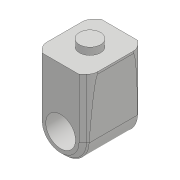
# Autodesk Inventor part: link4
Saved by Autodesk Inventor 2018 (Build 220112000, 112)
## iProperties
Created: 2018-02-01
Part Number: link4
Material: Generic
Document SubType Name: Modeling
Designer: Clevo
Density: 1 g/cm^3
Appearance: Default
Author: Clevo
Autodesk Inventor part; units mm, degrees
ref_plane "YZ Plane" through (0, 0, 0) normal (1, 0, 0) x (0, 1, 0)
ref_plane "XZ Plane" through (0, 0, 0) normal (0, 1, 0) x (-1, 0, 0)
ref_plane "XY Plane" through (0, 0, 0) normal (0, 0, 1) x (1, 0, 0)
sketch "Sketch1" plane through (0, 0, 0) normal (0, 1, 0) x (-1, 0, 0)
  line L0 (12.25, 22.5) -> (-12.25, 22.5)
  line L1 (-12.25, 22.5) -> (-12.25, -22.5)
  line L2 (-12.25, -22.5) -> (12.25, -22.5)
  line L3 (12.25, -22.5) -> (12.25, 22.5)
  point P0 (0, 0)
  point P1 (12.25, 0)
  point P2 (0, 22.5)
  dimension "d0" = 24.5
  dimension "d1" = 45
  constraints: 8 end point, 2 midpoint, 2 parallel, 1 horizontal, 1 horizontal alignment, 1 perpendicular, 1 vertical alignment
  measures "d0" distance of L2.end L1.end
  measures "d1" distance of L1.end L0.end
extrude "Extrusion1" add sketch "Sketch1" along normal blind 1.95
sketch "Sketch2" plane through (0, 1.95, 0) normal (0, 1, 0) x (1, 0, 0)
  line L0 (-10, 1.25) -> (10, 1.25)
  line L1 (10, 1.25) -> (10, -17.25)
  line L2 (10, -17.25) -> (-10, -17.25)
  line L3 (-10, -17.25) -> (-10, 1.25)
  line L4 (-12.25, -22.5) -> (12.25, -22.5) projected
  line L5 (12.25, -22.5) -> (12.25, 22.5) projected
  line L6 (12.25, 22.5) -> (-12.25, 22.5) projected
  line L7 (-12.25, 22.5) -> (-12.25, -22.5) projected
  line L8 (-7, -17.25) -> (7, -17.25)
  line L9 (7, -17.25) -> (7, -22.5)
  line L10 (7, -22.5) -> (-7, -22.5)
  line L11 (-7, -22.5) -> (-7, -17.25)
  line L12 (-12.25, -22.5) -> (12.25, -22.5) projected
  point P0 (0, 0)
  dimension "d4" = 2.25
  dimension "d5" = 20
  dimension "d6" = 2.25
  dimension "d7" = 5.25
  dimension "d8" = 5.25
  dimension "d9" = 14
  dimension "d10" = 5.25
  dimension "d11" = 18.5
  constraints: 16 end point, 4 parallel, 2 horizontal, 2 perpendicular, 1 collinear, 1 point on line
  measures "d4" distance between parallel lines of L7 L3
  measures "d5" distance of L0.start L0.end
  measures "d6" distance between parallel lines of L5 L1
  measures "d7" distance of L8.end L9.end
  measures "d8" distance between parallel lines of L7 L11
  measures "d9" distance between parallel lines of L9 L11
  measures "d10" distance between parallel lines of L5 L9
  measures "d11" distance of L0.end L1.end
extrude "Extrusion2" cut sketch "Sketch2" against normal up to surface (1.95 mm away) contours L0 L1 L2 L3 | L2 L9 L4 L11
sketch "Sketch3" plane through (0, 1.95, 0) normal (0, 1, 0) x (1, 0, 0)
  line L0 (-7, -22.5) -> (-7, -17.25) projected
  line L1 (-7, -17.25) -> (-10, -17.25) projected
  line L2 (-10, -17.25) -> (-10, 1.25) projected
  line L3 (-10, 1.25) -> (10, 1.25) projected
  line L4 (10, 1.25) -> (10, -17.25) projected
  line L5 (10, -17.25) -> (7, -17.25) projected
  line L6 (7, -17.25) -> (7, -22.5) projected
  line L7 (7, -22.5) -> (12.25, -22.5) projected
  line L8 (12.25, -22.5) -> (12.25, 22.5) projected
  line L9 (12.25, 22.5) -> (-12.25, 22.5) projected
  line L10 (-12.25, 22.5) -> (-12.25, -22.5) projected
  line L11 (-12.25, -22.5) -> (-7, -22.5) projected
  point P0 (0, 0)
  point P1 (-10.25, -20.305)
  point P2 (10.25, -20.305)
  dimension "d14" = 20.5
  dimension "d15" = 2
  dimension "d16" = 2.195
  dimension "d17" = 2
  constraints: 1 horizontal alignment
  measures "d14" distance of point (10.25, -20.305) point (-10.25, -20.305)
  measures "d15" distance from line of L8 point (10.25, -20.305)
  measures "d16" distance from line of L11 point (-10.25, -20.305)
  measures "d17" distance from line of L10 point (-10.25, -20.305)
hole "Hole1" at (-10.25, 1.95, 20.305) at (10.25, 1.95, 20.305) direction (0, -1, 0) diameter 2.4 end through all clearance for "Flat Head Machine Screw" size "M2" standard "Ansi Metric M Profile"
sketch "Sketch4" plane through (0, 1.95, 0) normal (0, 1, 0) x (1, 0, 0)
  circle A0 centre (-10.25, -20.305) radius 1.2 projected
  circle A1 centre (10.25, -20.305) radius 1.2 projected
  line L0 (-7, -22.5) -> (-7, -17.25) projected
  line L1 (-7, -17.25) -> (-10, -17.25) projected
  line L2 (-10, -17.25) -> (-10, 1.25) projected
  line L3 (-10, 1.25) -> (10, 1.25) projected
  line L4 (10, 1.25) -> (10, -17.25) projected
  line L5 (10, -17.25) -> (7, -17.25) projected
  line L6 (7, -17.25) -> (7, -22.5) projected
  line L7 (7, -22.5) -> (12.25, -22.5) projected
  line L8 (12.25, -22.5) -> (12.25, 22.5) projected
  line L9 (12.25, 22.5) -> (-12.25, 22.5) projected
  line L10 (-12.25, 22.5) -> (-12.25, -22.5) projected
  line L11 (-12.25, -22.5) -> (-7, -22.5) projected
  point P0 (0, 0)
  point P1 (-10.25, 4.15)
  point P2 (10.25, 4.15)
  dimension "d25" = 20.5
  dimension "d26" = 26.65
  dimension "d27" = 2
  dimension "d28" = 2
  constraints: 1 horizontal alignment
  measures "d25" distance of point (10.25, 4.15) point (-10.25, 4.15)
  measures "d26" distance from line of L11 point (-10.25, 4.15)
  measures "d27" distance from line of L10 point (-10.25, 4.15)
  measures "d28" distance from line of L8 point (10.25, 4.15)
hole "Hole2" at (-10.25, 1.95, -4.15) at (10.25, 1.95, -4.15) direction (0, -1, 0) diameter 2.4 end through all clearance for "Flat Head Machine Screw" size "M2" standard "Ansi Metric M Profile"
fillet "Fillet1" radius 0.5 2 edges at (7, 0.975, 17.25) (-7, 0.975, 17.25)
sketch "Sketch5" plane through (0, 1.95, 0) normal (0, 1, 0) x (1, 0, 0)
  circle A0 centre (-10.25, 4.15) radius 1.2 projected
  circle A1 centre (10.25, 4.15) radius 1.2 projected
  circle A2 centre (-10.25, -20.305) radius 1.2 projected
  circle A3 centre (10.25, -20.305) radius 1.2 projected
  arc A4 (-7, -17.75) -> (-7.5, -17.25) centre (-7.5, -17.75) ccw projected
  line L0 (-7.5, -17.25) -> (-10, -17.25) projected
  line L1 (-10, -17.25) -> (-10, 1.25) projected
  line L2 (-10, 1.25) -> (10, 1.25) projected
  line L3 (10, 1.25) -> (10, -17.25) projected
  line L4 (10, -17.25) -> (7.5, -17.25) projected
  arc A5 (7.5, -17.25) -> (7, -17.75) centre (7.5, -17.75) ccw projected
  line L5 (7, -17.75) -> (7, -22.5) projected
  line L6 (7, -22.5) -> (12.25, -22.5) projected
  line L7 (12.25, -22.5) -> (12.25, 22.5) projected
  line L8 (12.25, 22.5) -> (-12.25, 22.5) projected
  line L9 (-12.25, 22.5) -> (-12.25, -22.5) projected
  line L10 (-12.25, -22.5) -> (-7, -22.5) projected
  line L11 (-7, -22.5) -> (-7, -17.75) projected
  line L12 (-12.25, 22.5) -> (-12.25, -22.5) projected
  line L13 (12.25, -22.5) -> (12.25, 22.5) projected
  line L14 (-12.25, -22.5) -> (12.25, -22.5)
  line L15 (12.25, -22.5) -> (12.25, -4.5)
  line L16 (12.25, -4.5) -> (10, -4.5)
  line L17 (-12.25, -4.5) -> (-12.25, -22.5)
  line L18 (-10, -4.5) -> (-12.25, -4.5)
  line L19 (10, -4.5) -> (-10, -4.5)
  point P0 (0, 0)
  dimension "d37" = 18
  constraints: 12 end point, 4 parallel, 3 point on line, 1 horizontal, 1 perpendicular
  measures "d37" distance between parallel lines of L14 L16
extrude "Extrusion3" add sketch "Sketch5" along normal blind 5 contours L11 L10 L9 L18 L1 L0 A4 | A4 L0 L1 L19 L3 L4 A5 L5 L14 L11 | L5 A5 L4 L3 L16 L7 L6 | L18 L9 L8 L7 L16 L3 L2 L1
sketch "Sketch6" plane through (12.25, 0, 22.5) normal (1, 0, 0) x (0, 0, -1)
  line L0 (0, 0) -> (45, 0) projected
  line L1 (45, 0) -> (45, 6.95) projected
  line L2 (0, 6.95) -> (45, 6.95) projected
  line L3 (0, 0) -> (0, 6.95) projected
  line L4 (45, 0) -> (45, 6.95) projected
  line L5 (45, 6.95) -> (0, 6.95)
  line L6 (0, 6.95) -> (0, -32)
  line L7 (0, -32) -> (45, -32)
  line L8 (45, -32) -> (45, 6.95)
  line L9 (0, 0) -> (0, 6.95) projected
  line L10 (0, 0) -> (45, 0) projected
  line L11 (45, 0) -> (0, 0)
  line L12 (0, 0) -> (0, -32)
  line L13 (0, -32) -> (45, -32)
  line L14 (45, -32) -> (45, 0)
  point P0 (22.5, 0)
  dimension "d72" = 32
  constraints: 16 end point, 4 parallel, 2 horizontal, 2 perpendicular, 1 collinear
  measures "d72" distance between parallel lines of L0 L7
extrude "Extrusion4" add sketch "Sketch6" along normal blind 10
sketch "Sketch7" plane through (12.25, -32, -22.5) normal (0, -1, 0) x (1, 0, 0)
  line L0 (0, 45) -> (0, 0) projected
  line L1 (0, 0) -> (10, 0) projected
  line L2 (10, 45) -> (10, 0) projected
  line L3 (0, 45) -> (10, 45) projected
  line L4 (0, 0) -> (-24.5, 0) projected
  line L5 (0, 0) -> (-24.5, 0)
  line L6 (-24.5, 0) -> (-24.5, 45)
  line L7 (-24.5, 45) -> (0, 45)
  line L8 (0, 45) -> (0, 0)
  point P0 (-12.25, 22.5)
  dimension "d43" = 24.5
  constraints: 8 end point, 2 parallel, 1 collinear, 1 horizontal, 1 perpendicular
  measures "d43" distance of L0.end L5.end
extrude "Extrusion5" add sketch "Sketch7" along normal blind 1.15
sketch "Sketch8" plane through (12.25, -33.15, -22.5) normal (0, -1, 0) x (1, 0, 0)
  line L0 (-24.5, 0) -> (10, 0) projected
  line L1 (10, 0) -> (10, 45) projected
  line L2 (10, 45) -> (-24.5, 45) projected
  line L3 (-24.5, 45) -> (-24.5, 0) projected
  circle A0 centre (-12.25, 10) radius 10.5
  line L4 (-19.25, 45) -> (-5.25, 45) projected
  line L5 (-5, 45) -> (-19.5, 45)
  line L6 (-19.5, 45) -> (-19.5, 36)
  line L7 (-19.5, 36) -> (-5, 36)
  line L8 (-5, 36) -> (-5, 45)
  line L9 (-2.25, 21.25) -> (-22.25, 21.25)
  line L10 (-22.25, 21.25) -> (-22.25, 36)
  line L11 (-22.25, 36) -> (-2.25, 36)
  line L12 (-2.25, 36) -> (-2.25, 21.25)
  line L13 (-5, 21.25) -> (-19.5, 21.25)
  line L14 (-19.5, 21.25) -> (-19.5, 17.25)
  line L15 (-19.5, 17.25) -> (-5, 17.25)
  line L16 (-5, 17.25) -> (-5, 21.25)
  line L17 (-24.5, 0) -> (10, 0) projected
  line L18 (-24.5, 45) -> (0, 45)
  line L19 (0, 45) -> (0, 0)
  line L20 (0, 0) -> (-24.5, 0)
  line L21 (-24.5, 0) -> (-24.5, 45)
  point P0 (-12.25, 22.5)
  dimension "d46" = 10
  dimension "d47" = 21
  dimension "d48" = 14.5
  dimension "d49" = 20
  dimension "d50" = 14.5
  dimension "d51" = 24.5
  dimension "d52" = 5
  dimension "d53" = 5
  dimension "d54" = 2.25
  dimension "d55" = 2.25
  dimension "d56" = 5
  dimension "d57" = 5
  dimension "d58" = 9
  dimension "d59" = 14.75
  dimension "d60" = 4
  constraints: 32 end point, 8 parallel, 4 horizontal, 4 perpendicular, 4 point on line, 1 centre point, 1 vertical alignment
  measures "d46" distance from line of L0 A0.centre
  measures "d47" diameter of A0
  measures "d48" distance between parallel lines of L6 L8
  measures "d49" distance of L10.end L11.end
  measures "d50" distance of L14.end L15.end
  measures "d51" distance between parallel lines of L3 L19
  measures "d52" distance between parallel lines of L19 L16
  measures "d53" distance between parallel lines of L3 L14
  measures "d54" distance between parallel lines of L19 L12
  measures "d55" distance between parallel lines of L3 L10
  measures "d56" distance between parallel lines of L3 L6
  measures "d57" distance between parallel lines of L19 L8
  measures "d58" distance of L5.end L6.end
  measures "d59" distance of L9.end L10.end
  measures "d60" distance of L13.end L14.end
extrude "Extrusion6" cut sketch "Sketch8" against normal up to surface (1.15 mm away) contours A0 L0 | L0 A0 L14 L15 L16 | L8 L7 L6 L2 | L14 L9 L16 A0 | A0 L16 L15 L14 | L11 L12 L9 L10 L7
sketch "Sketch9" plane through (12.25, -33.15, -22.5) normal (0, -1, 0) x (1, 0, 0)
  line L0 (-5, 45) -> (-5, 36) projected
  line L1 (-5, 36) -> (-2.25, 36) projected
  line L2 (-2.25, 36) -> (-2.25, 21.25) projected
  line L3 (-2.25, 21.25) -> (-5, 21.25) projected
  line L4 (-5, 21.25) -> (-5, 17.5952) projected
  arc A0 (-9.0484, 0) -> (-5, 17.5952) centre (-12.25, 10) ccw projected
  line L5 (-9.0484, 0) -> (10, 0) projected
  line L6 (10, 0) -> (10, 45) projected
  line L7 (10, 45) -> (-5, 45) projected
  line L8 (-19.5, 36) -> (-19.5, 45) projected
  line L9 (-19.5, 45) -> (-24.5, 45) projected
  line L10 (-24.5, 45) -> (-24.5, 0) projected
  line L11 (-24.5, 0) -> (-15.4516, 0) projected
  arc A1 (-19.5, 17.5952) -> (-15.4516, 0) centre (-12.25, 10) ccw projected
  line L12 (-19.5, 17.5952) -> (-19.5, 21.25) projected
  line L13 (-19.5, 21.25) -> (-22.25, 21.25) projected
  line L14 (-22.25, 21.25) -> (-22.25, 36) projected
  line L15 (-22.25, 36) -> (-19.5, 36) projected
  circle A2 centre (-22.5, 18.35) radius 1.2 projected
  circle A3 centre (-2, 18.35) radius 1.2 projected
  circle A4 centre (-2, 42.805) radius 1.2 projected
  circle A5 centre (-22.5, 42.805) radius 1.2 projected
  line L16 (-2, 18.35) -> (-22.5, 18.35)
  line L17 (-22.5, 18.35) -> (-22.5, 39.05)
  line L18 (-22.5, 39.05) -> (-2, 39.05)
  line L19 (-2, 39.05) -> (-2, 18.35)
  point P0 (-12.25, 22.5)
  dimension "d63" = 20.7
  constraints: 8 end point, 2 parallel, 1 horizontal, 1 perpendicular, 1 point on line
  measures "d63" distance of L16.end L17.end
hole "Hole3" at (-10.25, -33.15, -4.15) at (10.25, -33.15, -4.15) at (10.25, -33.15, 16.55) at (-10.25, -33.15, 16.55) direction (0, 1, 0) diameter 2.4 depth 8 tip angle 118 clearance for "Flat Head Machine Screw" size "M2" standard "Ansi Metric M Profile"
sketch "Sketch10" plane through (12.25, -33.15, -22.5) normal (0, -1, 0) x (1, 0, 0)
  circle A0 centre (-2, 39.05) radius 1.2 projected
  circle A1 centre (-2, 18.35) radius 1.2 projected
  line L0 (-5, 45) -> (-5, 36) projected
  line L1 (-5, 36) -> (-2.25, 36) projected
  line L2 (-2.25, 36) -> (-2.25, 21.25) projected
  line L3 (-2.25, 21.25) -> (-5, 21.25) projected
  line L4 (-5, 21.25) -> (-5, 17.5952) projected
  arc A2 (-9.0484, 0) -> (-5, 17.5952) centre (-12.25, 10) ccw projected
  line L5 (-9.0484, 0) -> (10, 0) projected
  line L6 (10, 0) -> (10, 45) projected
  line L7 (10, 45) -> (-5, 45) projected
  circle A3 centre (-22.5, 18.35) radius 1.2 projected
  circle A4 centre (-22.5, 39.05) radius 1.2 projected
  line L8 (-19.5, 36) -> (-19.5, 45) projected
  line L9 (-19.5, 45) -> (-24.5, 45) projected
  line L10 (-24.5, 45) -> (-24.5, 0) projected
  line L11 (-24.5, 0) -> (-15.4516, 0) projected
  arc A5 (-19.5, 17.5952) -> (-15.4516, 0) centre (-12.25, 10) ccw projected
  line L12 (-19.5, 17.5952) -> (-19.5, 21.25) projected
  line L13 (-19.5, 21.25) -> (-22.25, 21.25) projected
  line L14 (-22.25, 21.25) -> (-22.25, 36) projected
  line L15 (-22.25, 36) -> (-19.5, 36) projected
  line L16 (10, 0) -> (10, 45) projected
  line L17 (-24.5, 0) -> (-24.5, 45) projected
  line L18 (10, 0) -> (-24.5, 0)
  line L19 (-24.5, 0) -> (-24.5, 45)
  line L20 (-24.5, 45) -> (10, 45)
  line L21 (10, 45) -> (10, 0)
  arc A6 (-19.5, 17.5952) -> (-15.4516, 0) centre (-12.25, 10) ccw projected
  circle A7 centre (-12.25, 10) radius 10.5
  point P0 (-12.25, 22.5)
  constraints: 8 end point, 2 parallel, 1 coincident, 1 horizontal, 1 perpendicular, 3 other
extrude "Extrusion7" add sketch "Sketch10" along normal blind 5
sketch "Sketch11" plane through (12.25, -38.15, -22.5) normal (0, -1, 0) x (1, 0, 0)
  line L0 (-9.0484, 0) -> (10, 0) projected
  line L1 (10, 0) -> (10, 45) projected
  line L2 (10, 45) -> (-24.5, 45) projected
  line L3 (-24.5, 45) -> (-24.5, 0) projected
  line L4 (-24.5, 0) -> (-15.4516, 0) projected
  arc A0 (-15.4516, 0) -> (-9.0484, 0) centre (-12.25, 10) ccw projected
  arc A1 (-19.5, 17.5952) -> (-15.4516, 0) centre (-12.25, 10) ccw projected
  circle A2 centre (-12.25, 10) radius 10.5
  point P0 (-12.25, 22.5)
  constraints: 1 coincident, 3 other
extrude "Extrusion8" cut sketch "Sketch11" against normal up to surface (5 mm away) contours A0 A1 A2
sketch "Sketch12" plane through (-12.25, 0, -22.5) normal (-1, 0, 0) x (0, 0, 1)
  line L0 (-6.0754, -39.5109) -> (50.3226, -39.5109)
  line L1 (50.3226, -39.5109) -> (50.3226, 16.733)
  line L2 (50.3226, 16.733) -> (-6.0754, 16.733)
  line L3 (-6.0754, 16.733) -> (-6.0754, -39.5109)
  point P0 (22.5, 0)
  constraints: 8 end point, 2 parallel, 1 horizontal, 1 perpendicular
extrude "Extrusion9" cut sketch "Sketch12" against normal blind 12.25
sketch "Sketch13" plane through (0, 0, 0) normal (0, -1, 0) x (1, 0, 0)
  arc A0 (3.2016, -22.5) -> (0, -2) centre (0, -12.5) ccw projected
  circle A1 centre (0, -12.5) radius 4
  point P0 (0, 0)
  dimension "d80" = 8
  constraints: 1 centre point, 1 coincident
  measures "d80" diameter of A1
extrude "Extrusion10" cut sketch "Sketch13" against normal blind 4.5
sketch "Sketch14" plane through (12.25, 0, 22.5) normal (-1, 0, 0) x (0, 0, 1)
  line L0 (0, 0) -> (-45, 0) projected
  line L1 (-45, -32) -> (-45, 0) projected
  line L2 (0, -32) -> (-45, -32) projected
  line L3 (0, 0) -> (0, -32) projected
  point P0 (-22.5, 0)
extrude "Extrusion11" cut sketch "Sketch14" against normal blind 0.2
sketch "Sketch15" plane through (0, 6.95, 0) normal (0, 1, 0) x (1, 0, 0)
  arc A0 (0, 8.5) -> (0, 16.5) centre (0, 12.5) ccw projected
  circle A1 centre (0, 12.5) radius 10.5
  point P0 (0, 0)
  dimension "d86" = 21
  constraints: 1 centre point, 1 coincident
  measures "d86" diameter of A1
extrude "Extrusion12" cut sketch "Sketch15" against normal up to surface (6.95 mm away)
sketch "Sketch16" plane through (22.25, -38.15, -22.5) normal (0, 0, -1) x (-1, 0, 0)
  line L0 (19.0484, 45.1) -> (0, 45.1) projected
  line L1 (0, 45.1) -> (0, 0) projected
  line L2 (19.0484, 0) -> (0, 0) projected
  line L3 (19.0484, 6.15) -> (9.8, 6.15) projected
  line L4 (9.8, 6.15) -> (9.8, 38.15) projected
  line L5 (9.8, 38.15) -> (19.0484, 38.15) projected
  line L6 (22.25, 45.1) -> (22.25, 40.1) projected
  line L7 (0, 0) -> (22.25, 0)
  line L8 (22.25, 0) -> (22.25, 45.1)
  line L9 (22.25, 45.1) -> (0, 45.1)
  line L10 (0, 45.1) -> (0, 0)
  line L11 (19.0484, 38.15) -> (19.0484, 45.1) projected
  line L12 (19.0484, 0) -> (19.0484, 6.15) projected
  point P0 (22.25, 38.15)
  constraints: 8 end point, 2 parallel, 1 horizontal, 1 perpendicular
extrude "Extrusion13" add sketch "Sketch16" along normal blind 8
sketch "Sketch17" plane through (7, 0, 22.5) normal (0, 0, 1) x (1, 0, 0)
  line L0 (0, 0) -> (5.45, 0) projected
  line L1 (5.45, 0) -> (5.45, -32) projected
  line L2 (5.45, -32) -> (0.25, -32) projected
  line L3 (0.25, -32) -> (0.25, -33.15) projected
  line L4 (0.25, -33.15) -> (-7, -33.15) projected
  line L5 (-7, -33.15) -> (-7, -38.15) projected
  line L6 (15.25, -38.15) -> (-7, -38.15) projected
  line L7 (15.25, 6.95) -> (15.25, -38.15) projected
  line L8 (-7, 6.95) -> (15.25, 6.95) projected
  line L9 (-7, 6.95) -> (-7, 1.95) projected
  line L10 (-7, 1.95) -> (0, 1.95) projected
  line L11 (0, 1.95) -> (0, 0) projected
  line L12 (-7, 6.95) -> (15.25, 6.95) projected
  line L13 (-7, -38.15) -> (-7, -33.15) projected
  line L14 (15.25, 6.95) -> (-7, 6.95)
  line L15 (-7, 6.95) -> (-7, -38.15)
  line L16 (-7, -38.15) -> (15.25, -38.15)
  line L17 (15.25, -38.15) -> (15.25, 6.95)
  point P0 (-7, 0)
  constraints: 8 end point, 2 parallel, 1 horizontal, 1 perpendicular
extrude "Extrusion14" add sketch "Sketch17" along normal blind 5
sketch "Sketch18" plane through (12.25, -38.15, -22.5) normal (0, -1, 0) x (1, 0, 0)
  line L0 (-12.25, 50) -> (-12.25, 20.5) projected
  arc A0 (-9.0484, 0) -> (-12.25, 20.5) centre (-12.25, 10) ccw projected
  line L1 (-9.0484, 0) -> (-12.25, 0) projected
  line L2 (-12.25, 0) -> (-12.25, -8) projected
  line L3 (10, -8) -> (-12.25, -8) projected
  line L4 (10, 50) -> (10, -8) projected
  line L5 (-12.25, 50) -> (10, 50) projected
  circle A1 centre (-2, 39.05) radius 1.2 projected
  circle A2 centre (-2, 18.35) radius 1.2 projected
  line L6 (-12.25, 21.25) -> (-12.25, 20.5) projected
  circle A3 centre (-12.25, 10) radius 10.5
  point P0 (-12.25, 22.5)
  constraints: 1 coincident, 1 vertical alignment, 2 other
extrude "Extrusion15" cut sketch "Sketch18" against normal up to surface (45.1 mm away) contours A0 L1 L2 A3 | L2 L1 A3
sketch "Sketch19" plane through (22.25, -38.15, -22.5) normal (0, 0, 1) x (1, 0, 0)
  line L0 (-19.0484, 38.15) -> (-19.0484, 6.15) projected
  line L1 (-19.0484, 6.15) -> (-9.8, 6.15) projected
  line L2 (-9.8, 6.15) -> (-9.8, 38.15) projected
  line L3 (-9.8, 38.15) -> (-19.0484, 38.15) projected
  line L4 (-9.8, 38.15) -> (-39.7398, 38.15)
  line L5 (-39.7398, 38.15) -> (-39.7398, 6.15)
  line L6 (-39.7398, 6.15) -> (-9.8, 6.15)
  line L7 (-9.8, 6.15) -> (-9.8, 38.15)
  point P0 (-22.25, 38.15)
  constraints: 8 end point, 2 parallel, 1 collinear, 1 horizontal, 1 perpendicular
extrude "Extrusion16" cut sketch "Sketch19" against normal blind 0.2
sketch "Sketch20" plane through (7, 0, 22.5) normal (0, 0, -1) x (-1, 0, 0)
  line L0 (-0.25, -33.15) -> (7, -33.15) projected
  line L1 (7, 1.95) -> (7, -33.15) projected
  line L2 (7, 1.95) -> (0, 1.95) projected
  line L3 (0, 1.95) -> (0, 0) projected
  line L4 (0, 0) -> (-5.45, 0) projected
  line L5 (-5.45, 0) -> (-5.45, -32) projected
  line L6 (-5.45, -32) -> (-0.25, -32) projected
  line L7 (-0.25, -32) -> (-0.25, -33.15) projected
  point P0 (7, 0)
extrude "Extrusion17" cut sketch "Sketch20" against normal blind 0.2
chamfer "Chamfer1" distance 2.5 angle 45 1 edges at (12.45, -16, -22.7)
fillet "Fillet7" radius 1.5 1 edges at (12.45, -16, 22.7)
fillet "Fillet8" radius 0.5 2 edges at (7.25, -32.575, -1.25) (7.25, -32.575, 13.5)
mirror "Mirror1" about plane through (0, -11.389, -0.3764) normal (-1, 0, 0)
sketch "Sketch25" plane through (0, 6.95, 0) normal (0, 1, 0) x (1, 0, 0)
  line L0 (-10, 1.25) -> (10, 1.25) projected
  line L1 (10, 1.25) -> (10, -4.5) projected
  line L2 (-10, -4.5) -> (10, -4.5) projected
  line L3 (-10, 1.25) -> (-10, -4.5) projected
  circle A0 centre (0, 12.5) radius 10.5 projected
  circle A1 centre (-10.25, -20.305) radius 1.2 projected
  circle A2 centre (-10.25, 4.15) radius 1.2 projected
  line L4 (22.25, 30.5) -> (-22.25, 30.5) projected
  line L5 (-22.25, -27.5) -> (-22.25, 30.5) projected
  line L6 (22.25, -27.5) -> (-22.25, -27.5) projected
  line L7 (22.25, -27.5) -> (22.25, 30.5) projected
  circle A3 centre (10.25, 4.15) radius 1.2 projected
  circle A4 centre (10.25, -20.305) radius 1.2 projected
  point P0 (0, 0)
extrude "Extrusion19" cut sketch "Sketch25" against normal blind 1.8
sketch "Sketch26" plane through (12.25, -38.15, -22.5) normal (0, -1, 0) x (1, 0, 0)
  line L0 (10, -8) -> (-34.5, -8) projected
  line L1 (10, 50) -> (10, -8) projected
  line L2 (10, 50) -> (-34.5, 50) projected
  line L3 (-34.5, 50) -> (-34.5, -8) projected
  circle A0 centre (-22.5, 18.35) radius 1.2 projected
  circle A1 centre (-22.5, 39.05) radius 1.2 projected
  circle A2 centre (-12.25, 10) radius 10.5 projected
  circle A3 centre (-2, 39.05) radius 1.2 projected
  circle A4 centre (-2, 18.35) radius 1.2 projected
  point P0 (-12.25, 22.5)
extrude "Extrusion20" cut sketch "Sketch26" against normal blind 1.8
sketch "Sketch27" plane through (7, 0, 27.5) normal (0, 0, 1) x (1, 0, 0)
  line L0 (11.0275, 5.15) -> (-25.0275, 5.15)
  line L1 (-25.0275, 5.15) -> (-25.0275, -36.35)
  line L2 (-25.0275, -36.35) -> (11.0275, -36.35)
  line L3 (11.0275, -36.35) -> (11.0275, 5.15)
  line L4 (-29.25, -36.35) -> (15.25, -36.35) projected
  line L5 (15.25, -36.35) -> (15.25, 5.15) projected
  line L6 (15.25, 5.15) -> (-29.25, 5.15) projected
  line L7 (-29.25, -36.35) -> (-29.25, 5.15) projected
  line L8 (-29.25, -36.35) -> (15.25, -36.35) projected
  point P0 (-7, 0)
  dimension "d133" = 36.055
  dimension "d134" = 4.2225
  dimension "d135" = 4.2225
  constraints: 8 end point, 2 collinear, 2 parallel, 1 horizontal, 1 perpendicular
  measures "d133" distance of L0.start L0.end
  measures "d134" distance between parallel lines of L7 L1
  measures "d135" distance between parallel lines of L5 L3
extrude "Extrusion21" cut sketch "Sketch27" against normal up to surface (58 mm away) contours L6 L5 L4 L3 | L1 L4 L7 L6
sketch "Sketch29" plane through (12.25, -36.35, -22.5) normal (0, -1, 0) x (1, 0, 0)
  line L0 (-30.2775, 50) -> (-30.2775, -8) projected
  line L1 (5.7775, -8) -> (-30.2775, -8) projected
  line L2 (5.7775, -8) -> (5.7775, 50) projected
  line L3 (-30.2775, 50) -> (5.7775, 50) projected
  circle A0 centre (-12.25, 10) radius 10.5 projected
  circle A1 centre (-2, 18.35) radius 1.2 projected
  circle A2 centre (-2, 39.05) radius 1.2 projected
  circle A3 centre (-22.5, 39.05) radius 1.2 projected
  circle A4 centre (-22.5, 18.35) radius 1.2 projected
  line L4 (5.7775, 50) -> (5.7775, -8) projected
  line L5 (-30.2775, -8) -> (-30.2775, 50) projected
  line L6 (5.7775, 50) -> (-30.2775, 50)
  line L7 (-30.2775, 50) -> (-30.2775, 10)
  line L8 (-30.2775, 10) -> (5.7775, 10)
  line L9 (5.7775, 10) -> (5.7775, 50)
  circle A5 centre (-12.25, 10) radius 18.0275
  point P0 (-12.25, 22.5)
  constraints: 8 end point, 2 parallel, 1 centre point, 1 coincident, 1 horizontal, 1 midpoint, 1 perpendicular, 1 point on line, 1 tangent
extrude "Extrusion22" cut sketch "Sketch29" against normal up to surface (41.5 mm away) contours L3 L2 A5 L0 | A5 L8 A0 | L8 A0 A5 L1 | L8 A0 | A0 L8 | L1 A5 | A1 | A2 | A3 | A4 keep common part
sketch "Sketch30" plane through (12.25, -36.35, -22.5) normal (0, -1, 0) x (1, 0, 0)
  line L0 (-11.2546, -8) -> (-13.2454, -8) projected
  circle A0 centre (-22.5, 18.35) radius 1.2 projected
  circle A1 centre (-22.5, 39.05) radius 1.2 projected
  circle A2 centre (-2, 39.05) radius 1.2 projected
  circle A3 centre (-2, 18.35) radius 1.2 projected
  circle A4 centre (-12.25, 10) radius 10.5 projected
  arc A5 (-11.2546, -8) -> (5.7775, 10) centre (-12.25, 10) ccw projected
  line L1 (5.7775, 10) -> (5.7775, 50) projected
  line L2 (-30.2775, 50) -> (5.7775, 50) projected
  line L3 (-30.2775, 50) -> (-30.2775, 10) projected
  arc A6 (-30.2775, 10) -> (-13.2454, -8) centre (-12.25, 10) ccw projected
  line L4 (-11.2546, -8) -> (-13.2454, -8) projected
  arc A7 (-30.2775, 10) -> (-13.2454, -8) centre (-12.25, 10) ccw projected
  arc A8 (5.7775, 10) -> (-13.2454, -8) centre (-12.25, 10) ccw
  arc A9 (-11.2546, -8) -> (5.7775, 10) centre (-12.25, 10) ccw
  arc A10 (-13.2454, -8) -> (-11.2546, -8) centre (-12.25, 10) ccw
  point P0 (-12.25, 22.5)
  constraints: 8 point on circle, 3 centre point, 3 end point, 1 coincident
extrude "Extrusion23" add sketch "Sketch30" against normal up to surface (41.5 mm away) contours A10 L0
chamfer "Chamfer2" distance 5 angle 45 8 edges at (18.0275, -36.35, 7.5) (-13.0946, -36.35, -24.8905) (13.0946, -36.35, -24.8905) (-18.0275, -36.35, 7.5) (-13.0946, 5.15, -24.8905) (13.0946, 5.15, -24.8905) (18.0275, 5.15, 7.5) (-18.0275, 5.15, 7.5)
fillet "Fillet9" radius 8 8 edges at (18.0275, -31.35, 7.5) (-13.0946, -31.35, -24.8905) (13.0946, -31.35, -24.8905) (-18.0275, -31.35, 7.5) (-13.0946, 0.15, -24.8905) (13.0946, 0.15, -24.8905) (-18.0275, 0.15, 7.5) (18.0275, 0.15, 7.5)
sketch "Sketch32" plane through (12.25, -36.35, -22.5) normal (0, -1, 0) x (1, 0, 0)
  line L0 (-30.2775, 50) -> (-27.9344, 50) projected
  line L1 (-27.9344, 50) -> (-30.2775, 50) projected
  line L2 (-25.2775, 50) -> (-27.9344, 50) projected
  line L3 (-25.2775, 50) -> (0.7775, 50) projected
  line L4 (3.4344, 50) -> (0.7775, 50) projected
  line L5 (5.7775, 50) -> (3.4344, 50) projected
  line L6 (3.4344, 50) -> (5.7775, 50) projected
  line L7 (0.7775, 50) -> (3.4344, 50) projected
  line L8 (0.7775, 50) -> (-25.2775, 50) projected
  line L9 (-27.9344, 50) -> (-25.2775, 50) projected
  line L10 (0.7775, 50) -> (0.7775, 10) projected
  line L11 (-25.2775, 50) -> (0.7775, 50) projected
  line L12 (-25.2775, 10) -> (-25.2775, 50) projected
  arc A0 (-25.2775, 10) -> (0.7775, 10) centre (-12.25, 10) ccw projected
  circle A1 centre (-22.5, 18.35) radius 1.2 projected
  circle A2 centre (-22.5, 39.05) radius 1.2 projected
  circle A3 centre (-2, 39.05) radius 1.2 projected
  circle A4 centre (-2, 18.35) radius 1.2 projected
  circle A5 centre (-12.25, 10) radius 10.5 projected
  circle A6 centre (-12.25, 10) radius 10.5 projected
  circle A7 centre (-12.25, 10) radius 16.5
  line L13 (-30.2775, 50) -> (-28.7382, 9.3752)
  line L14 (5.7775, 50) -> (5.7775, 10) projected
  line L15 (5.7775, 50) -> (4.2382, 9.3752)
  line L16 (-35.1798, -12.0066) -> (14.7173, -12.0066)
  line L17 (14.7173, -12.0066) -> (14.7173, 50)
  line L18 (14.7173, 50) -> (5.7775, 50)
  line L19 (-35.1798, 50) -> (-35.1798, -12.0066)
  line L20 (-30.2775, 50) -> (-35.1798, 50)
  line L21 (5.7775, 50) -> (-30.2775, 50)
  point P0 (-12.25, 22.5)
  dimension "d147" = 33
  constraints: 16 end point, 4 parallel, 2 point on circle, 2 tangent, 1 centre point, 1 coincident, 1 horizontal, 1 perpendicular, 1 point on line
  measures "d147" diameter of A7
extrude "Extrusion24" cut sketch "Sketch32" against normal up to surface (41.5 mm away) contours L13 A7 L15 L18 L17 L16 L19 L20
sketch "Sketch36" plane through (7, 0, 27.5) normal (0, 0, 1) x (1, 0, 0)
  arc A0 (-22.6844, 2.4931) -> (-25.0275, -3.1637) centre (-17.0275, -3.1637) ccw projected
  line L0 (-25.0275, -3.1637) -> (-25.0275, -28.0363) projected
  arc A1 (-25.0275, -28.0363) -> (-22.6844, -33.6931) centre (-17.0275, -28.0363) ccw projected
  line L1 (-20.0275, -36.35) -> (-22.6844, -33.6931) projected
  line L2 (-20.0275, -36.35) -> (6.0275, -36.35) projected
  line L3 (8.6844, -33.6931) -> (6.0275, -36.35) projected
  arc A2 (8.6844, -33.6931) -> (11.0275, -28.0363) centre (3.0275, -28.0363) ccw projected
  line L4 (11.0275, -28.0363) -> (11.0275, -3.1637) projected
  arc A3 (11.0275, -3.1637) -> (8.6844, 2.4931) centre (3.0275, -3.1637) ccw projected
  line L5 (6.0275, 5.15) -> (8.6844, 2.4931) projected
  line L6 (6.0275, 5.15) -> (-20.0275, 5.15) projected
  line L7 (-22.6844, 2.4931) -> (-20.0275, 5.15) projected
  circle A4 centre (-6.9725, -15.6) radius 12.5
  line L8 (-19.4725, -28.1) -> (5.5275, -28.1)
  line L9 (5.5275, -28.1) -> (5.5275, -3.1)
  line L10 (5.5275, -3.1) -> (-19.4725, -3.1)
  line L11 (-19.4725, -3.1) -> (-19.4725, -28.1)
  line L12 (-19.5225, -28.15) -> (5.5775, -28.15)
  line L13 (5.5775, -28.15) -> (5.5775, -3.05)
  line L14 (5.5775, -3.05) -> (-19.5225, -3.05)
  line L15 (-19.5225, -3.05) -> (-19.5225, -28.15)
  point P0 (-7, 0)
  dimension "d161" = 20.75
  dimension "d162" = 18
  dimension "d163" = 25
  dimension "d164" = 0.05
  constraints: 16 end point, 4 parallel, 4 tangent, 2 perpendicular, 1 centre point, 1 coincident, 1 horizontal, 3 other
  measures "d161" distance from line of L2 point (-6.973, -15.6)
  measures "d162" distance from line of L4 point (-6.973, -15.6)
  measures "d163" diameter of A4
  measures "d164" distance between parallel lines of L11 L15
extrude "Extrusion27" cut sketch "Sketch36" against normal blind 7 contours A4 | L9 L8 A4 | A4 L10 L9 | A4 L11 L10 | L8 L11 A4 | L15 L14 L13 L12
sketch "Sketch37" plane through (7, 0, 27.5) normal (0, 0, 1) x (1, 0, 0)
  line L0 (5.5775, -3.05) -> (5.5775, -28.15) projected
  line L1 (5.5775, -28.15) -> (-19.5225, -28.15) projected
  line L2 (-19.5225, -28.15) -> (-19.5225, -3.05) projected
  line L3 (-19.5225, -3.05) -> (5.5775, -3.05) projected
  arc A0 (-22.6844, 2.4931) -> (-25.0275, -3.1637) centre (-17.0275, -3.1637) ccw projected
  line L4 (-25.0275, -3.1637) -> (-25.0275, -28.0363) projected
  arc A1 (-25.0275, -28.0363) -> (-22.6844, -33.6931) centre (-17.0275, -28.0363) ccw projected
  line L5 (-20.0275, -36.35) -> (-22.6844, -33.6931) projected
  line L6 (-20.0275, -36.35) -> (6.0275, -36.35) projected
  line L7 (8.6844, -33.6931) -> (6.0275, -36.35) projected
  arc A2 (8.6844, -33.6931) -> (11.0275, -28.0363) centre (3.0275, -28.0363) ccw projected
  line L8 (11.0275, -28.0363) -> (11.0275, -3.1637) projected
  arc A3 (11.0275, -3.1637) -> (8.6844, 2.4931) centre (3.0275, -3.1637) ccw projected
  line L9 (6.0275, 5.15) -> (8.6844, 2.4931) projected
  line L10 (6.0275, 5.15) -> (-20.0275, 5.15) projected
  line L11 (-22.6844, 2.4931) -> (-20.0275, 5.15) projected
  point P0 (-7, 0)
extrude "Extrusion28" add sketch "Sketch37" along normal blind 1.5
sketch "Sketch41" plane through (0, 5.15, 0) normal (0, 1, 0) x (1, 0, 0)
  arc A0 (13.0275, 12.5) -> (-13.0275, 12.5) centre (0, 12.5) ccw projected
  line L0 (-13.0275, -29) -> (-13.0275, 12.5) projected
  line L1 (13.0275, -29) -> (-13.0275, -29) projected
  line L2 (13.0275, 12.5) -> (13.0275, -29) projected
  circle A1 centre (0, 12.5) radius 10.5 projected
  line L3 (-10, 1.25) -> (-10, -4.5) projected
  line L4 (10, 1.25) -> (-10, 1.25) projected
  line L5 (10, -4.5) -> (10, 1.25) projected
  line L6 (-10, -4.5) -> (10, -4.5) projected
  circle A2 centre (10.25, -20.305) radius 1.2 projected
  circle A3 centre (10.25, 4.15) radius 1.2 projected
  circle A4 centre (-10.25, 4.15) radius 1.2 projected
  circle A5 centre (-10.25, -20.305) radius 1.2 projected
  line L7 (-10, -13.75) -> (10, -13.75)
  line L8 (10, -13.75) -> (10, 1.25)
  line L9 (10, 1.25) -> (-10, 1.25)
  line L10 (-10, 1.25) -> (-10, -13.75)
  point P0 (0, 0)
  dimension "d200" = 15
  constraints: 8 end point, 3 collinear, 2 parallel, 1 horizontal, 1 perpendicular
  measures "d200" distance of L9.end L7.start
extrude "Extrusion29" cut sketch "Sketch41" against normal up to surface (3.2 mm away) contours L6 L8 L7 L10
chamfer "Chamfer4" distance 1.5 angle 45 1 edges at (0, 5.15, 13.75)
sketch "Sketch44" plane through (0, 1.95, 0) normal (0, -1, 0) x (1, 0, 0)
  line L0 (-10, 13.75) -> (10, 13.75) projected
  line L1 (10, 13.75) -> (10, 17.25) projected
  line L2 (10, 17.25) -> (7.5, 17.25) projected
  arc A0 (7, 17.75) -> (7.5, 17.25) centre (7.5, 17.75) ccw projected
  line L3 (7, 17.75) -> (7, 22.7) projected
  line L4 (-7, 22.7) -> (7, 22.7) projected
  line L5 (-7, 17.75) -> (-7, 22.7) projected
  arc A1 (-7.5, 17.25) -> (-7, 17.75) centre (-7.5, 17.75) ccw projected
  line L6 (-10, 17.25) -> (-7.5, 17.25) projected
  line L7 (-10, 13.75) -> (-10, 17.25) projected
  circle A2 centre (-10.25, 20.305) radius 1.2 projected
  circle A3 centre (-10.25, -4.15) radius 1.2 projected
  arc A4 (12.45, 21.2) -> (10.95, 22.7) centre (10.95, 21.2) ccw projected
  line L8 (10.95, 22.7) -> (7, 22.7) projected
  line L9 (7, 22.7) -> (7, 17.75) projected
  arc A5 (7, 17.75) -> (7.5, 17.25) centre (7.5, 17.75) ccw projected
  line L10 (7.5, 17.25) -> (10, 17.25) projected
  line L11 (10, 17.25) -> (10, -1.25) projected
  line L12 (-10, -1.25) -> (10, -1.25) projected
  line L13 (-10, 17.25) -> (-10, -1.25) projected
  line L14 (-7.5, 17.25) -> (-10, 17.25) projected
  arc A6 (-7.5, 17.25) -> (-7, 17.75) centre (-7.5, 17.75) ccw projected
  line L15 (-7, 22.7) -> (-7, 17.75) projected
  line L16 (-10.95, 22.7) -> (-7, 22.7) projected
  arc A7 (-10.95, 22.7) -> (-12.45, 21.2) centre (-10.95, 21.2) ccw projected
  line L17 (-12.45, -20.2) -> (-12.45, 21.2) projected
  line L18 (-9.95, -22.7) -> (-12.45, -20.2) projected
  line L19 (-2.492, -22.7) -> (-9.95, -22.7) projected
  arc A8 (2.492, -22.7) -> (-2.492, -22.7) centre (0, -12.5) ccw projected
  line L20 (2.492, -22.7) -> (9.95, -22.7) projected
  line L21 (9.95, -22.7) -> (12.45, -20.2) projected
  line L22 (12.45, -20.2) -> (12.45, 21.2) projected
  circle A9 centre (10.25, -4.15) radius 1.2 projected
  circle A10 centre (10.25, 20.305) radius 1.2 projected
  point P0 (0, 0)
extrude "Extrusion30" add sketch "Sketch44" along normal up to surface (35.1 mm away) contours L7 L6 A1 L5 L4 L3 A0 L2 L1 L0 | L13 L12 L11 L1 L2 A0 L3 L8 A4 L22 L21 L20 A8 L19 L18 L17 A7 L16 L5 A1 L6 L7 | A2 | A3 | A9 | A10
sketch "Sketch45" plane through (0, 5.15, 0) normal (0, 1, 0) x (1, 0, 0)
  line L0 (-10, 1.25) -> (-10, -15.25) projected
  line L1 (10, 1.25) -> (-10, 1.25) projected
  line L2 (10, 1.25) -> (10, -15.25) projected
  line L3 (-10, -15.25) -> (10, -15.25) projected
  circle A0 centre (-10.25, -20.305) radius 1.2 projected
  circle A1 centre (-10.25, 4.15) radius 1.2 projected
  circle A2 centre (10.25, 4.15) radius 1.2 projected
  circle A3 centre (10.25, -20.305) radius 1.2 projected
  circle A4 centre (0, 12.5) radius 10.5 projected
  line L4 (13.0275, 12.5) -> (13.0275, -29) projected
  arc A5 (13.0275, 12.5) -> (-13.0275, 12.5) centre (0, 12.5) ccw projected
  line L5 (-13.0275, -29) -> (-13.0275, 12.5) projected
  line L6 (13.0275, -29) -> (-13.0275, -29) projected
  point P0 (0, 0)
extrude "Extrusion31" add sketch "Sketch45" against normal up to surface (41.5 mm away) contours L1 L2 L3 L0 | A0 | A1 | A2 | A3 | L4 L6 L5 A5
sketch "Sketch46" plane through (7, 0, 29) normal (0, 0, 1) x (1, 0, 0)
  line L0 (6.0275, -36.35) -> (8.6844, -33.6931) projected
  arc A0 (8.6844, -33.6931) -> (11.0275, -28.0363) centre (3.0275, -28.0363) ccw projected
  line L1 (11.0275, -28.0363) -> (11.0275, -3.1637) projected
  arc A1 (11.0275, -3.1637) -> (8.6844, 2.4931) centre (3.0275, -3.1637) ccw projected
  line L2 (8.6844, 2.4931) -> (6.0275, 5.15) projected
  line L3 (6.0275, 5.15) -> (-20.0275, 5.15) projected
  line L4 (-20.0275, 5.15) -> (-22.6844, 2.4931) projected
  arc A2 (-22.6844, 2.4931) -> (-25.0275, -3.1637) centre (-17.0275, -3.1637) ccw projected
  line L5 (-25.0275, -3.1637) -> (-25.0275, -28.0363) projected
  arc A3 (-25.0275, -28.0363) -> (-22.6844, -33.6931) centre (-17.0275, -28.0363) ccw projected
  line L6 (-22.6844, -33.6931) -> (-20.0275, -36.35) projected
  line L7 (-20.0275, -36.35) -> (6.0275, -36.35) projected
  line L8 (3.0275, -3.1637) -> (-17.0275, -3.1637)
  line L9 (-17.0275, -3.1637) -> (-17.0275, -28.0363)
  line L10 (-17.0275, -28.0363) -> (3.0275, -28.0363)
  line L11 (3.0275, -28.0363) -> (3.0275, -3.1637)
  line L12 (3.0275, -3.1637) -> (-17.0275, -28.0363) construction
  line L13 (-17.0275, -3.1637) -> (3.0275, -28.0363) construction
  circle A4 centre (-7, -15.6) radius 7.5
  point P0 (-7, 0)
  dimension "d226" = 15
  constraints: 12 end point, 2 coincident, 2 midpoint, 2 parallel, 1 centre point, 1 horizontal, 1 perpendicular
  measures "d226" diameter of A4
extrude "Extrusion32" add sketch "Sketch46" along normal blind 5 contours A4
equation "\"d4\" = d6"
equation "\"d8\" = d10"
equation "\"d15\" = d17"
equation "\"d27\" = d28"
equation "\"d52\" = d53"
equation "\"d54\" = d55"
equation "\"d56\" = d57"
equation "\"d134\" = d135"
body "Solid1"
